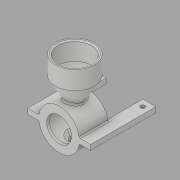
# Autodesk Inventor part: powderTurnRes
Saved by Autodesk Inventor 2017 (Build 210142000, 142)
## iProperties
Created: 2019-05-09
Part Number: powderTurnRes
Material: Generic
Document SubType Name: Modeling
Designer: Joe Sedutto
Density: 1 g/cm^3
Appearance: Default
Author: Joe Sedutto
Autodesk Inventor part; units mm, degrees
ref_plane "YZ Plane" through (0, 0, 0) normal (1, 0, 0) x (0, 1, 0)
ref_plane "XY Plane" through (0, 0, 0) normal (0, 0, 1) x (1, 0, 0)
sketch "Sketch1" plane through (0, 0, 0) normal (0, 0, 1) x (1, 0, 0)
  circle A0 centre (0, 0) radius 13.335
  circle A1 centre (0, 0) radius 19.685
  dimension "d0" = 26.67
  dimension "d1" = 6.35
  constraints: 2 centre point, 1 coincident
  measures "d0" diameter of A0
  measures "d1" radial gap between concentric circles of A0 A1
extrude "Extrusion1" add sketch "Sketch1" along normal blind 25.4
sketch "Sketch2" plane through (0, 0, 25.4) normal (0, 0, 1) x (1, 0, 0)
  circle A0 centre (0, 0) radius 13.335 projected
  circle A1 centre (0, 0) radius 19.685 projected
  circle A2 centre (0, 0) radius 12.065
  dimension "d4" = 1.27
  constraints: 1 centre point
  measures "d4" radial gap between concentric circles of A0 A2
extrude "Extrusion2" add sketch "Sketch2" along normal blind 2.54 contours A0 | A1
ref_plane "Work Plane1" through (0, 19.685, 0) normal (0, 1, 0) x (-1, 0, 0)
sketch "Sketch3" plane through (0, 19.685, 0) normal (0, 1, 0) x (-1, 0, 0)
  line L0 (-13.335, 0) -> (-13.335, 25.4) projected
  line L1 (0, 12.7) -> (-13.335, 12.7) construction
  line L2 (13.335, 0) -> (13.335, 25.4) projected
  line L3 (13.335, 12.7) -> (0, 12.7) construction
  point P0 (0, 0)
  constraints: 4 end point, 2 midpoint, 1 collinear, 1 horizontal
hole "Hole1" at (0, 19.685, 12.7) direction (0, -1, 0) diameter 6.35 depth 12.7 tip angle 118
ref_plane "Work Plane2" through (0, 0, 12.7) normal (0, 0, -1) x (-1, 0, 0)
sketch "Sketch4" plane through (0, 0, 12.7) normal (0, 0, -1) x (-1, 0, 0)
  line L0 (-3.175, 15.4915) -> (-16.228, 38.1)
  line L1 (-16.228, 38.1) -> (-18.768, 38.1)
  line L2 (-18.768, 38.1) -> (-5.715, 15.4915)
  line L3 (-5.715, 15.4915) -> (-3.175, 15.4915)
  circle A0 centre (0, 0) radius 19.685 projected
  line L4 (0, 19.685) -> (0, 34.1207) construction
  line L5 (-3.175, 12.9515) -> (-3.175, 19.4273) projected
  dimension "d15" = 2.54
  dimension "d16" = 38.1
  dimension "d17" = 30
  dimension "d18" = 2.54
  constraints: 10 end point, 2 parallel, 1 horizontal, 1 point on circle, 1 point on line, 1 vertical
  measures "d15" distance of L0.end L1.end
  measures "d16" distance from line of L1 point (0, 0)
  measures "d17" angle of L4 L2
  measures "d18" distance of L0.start L5.start
revolve "Revolution1" add sketch "Sketch4" angle 360 about axis through (0, 19.685, 12.7) along (0, 1, 0) contours L3 L2 A0 L0 | A0 L2 L1 L0
sketch "Sketch5" plane through (0, 38.1, 12.7) normal (0, 1, 0) x (1, 0, 0)
  circle A0 centre (0, 0) radius 18.768 projected
  circle A1 centre (0, 0) radius 16.228 projected
  point P0 (0, 12.7)
extrude "Extrusion3" add sketch "Sketch5" along normal blind 17.78
fillet "Fillet1" radius 1.27 1 edges at (-16.228, 55.88, 12.7)
fillet "Fillet2" radius 1.27 1 edges at (-7.3209, 18.273, 12.6991)
sketch "Sketch7" plane through (0, 0, 0) normal (0, 1, 0) x (-1, 0, 0)
  spline S0 degree 5 poles (0, 15.875) (0.3658, 15.875) (0.7269, 15.8223) (1.0689, 15.7198) (1.3811, 15.5769) (2.0115, 15.1917) (2.3108, 14.9286) (2.5556, 14.6369) (2.7488, 14.3276) (3.1275, 13.4883) (3.2362, 12.9391) (3.2299, 12.3842) (3.108, 11.8361) (2.6851, 10.9581) (2.4466, 10.6105) (2.1388, 10.2882) (1.7587, 10.0103) (0.8989, 9.6224) (0.4259, 9.4951) (-0.0811, 9.4669) (-0.5724, 9.5429) (-1.4458, 9.8363) (-1.8264, 10.0514) (-2.1489, 10.3127) (-2.4131, 10.6031) (-2.8482, 11.2413) (-3.0127, 11.5938) (-3.1209, 11.9589) (-3.175, 12.3292) (-3.175, 13.0561) (-3.1251, 13.4117) (-3.0253, 13.7627) (-2.8738, 14.1025) (-2.4642, 14.7367) (-2.2072, 15.0334) (-1.8916, 15.3023) (-1.5168, 15.5267) (-0.8852, 15.7566) (-0.6727, 15.8148) (-0.4518, 15.8549) (-0.2262, 15.875) (0, 15.875) knots 0 0 0 0 0 0 0.075674 0.075674 0.075674 0.075674 0.173825 0.173825 0.173825 0.173825 0.331664 0.331664 0.331664 0.331664 0.443615 0.443615 0.443615 0.443615 0.544209 0.544209 0.544209 0.544209 0.643845 0.643845 0.643845 0.643845 0.750428 0.750428 0.750428 0.750428 0.852775 0.852775 0.852775 0.852775 0.953216 0.953216 0.953216 0.953216 1 1 1 1 1 1
  spline S1 degree 5 poles (0, 17.145) (1.3934, 17.1441) (2.7891, 16.6018) (3.8921, 15.4994) (4.9888, 12.7159) (3.9096, 9.9248) (2.813, 8.8173) (0.0263, 7.709) (-2.7752, 8.7855) (-3.8891, 9.8896) (-4.9935, 12.6868) (-3.9033, 15.488) (-2.7986, 16.5982) (-1.3982, 17.1441) (0, 17.145) knots 0 0 0 0 0 0 0.249522 0.249522 0.249522 0.498935 0.498935 0.498935 0.749627 0.749627 0.749627 1 1 1 1 1 1
  point P0 (0, 0)
  dimension "d30" = 1.27
  constraints: 3 other
extrude "Extrusion5" cut sketch "Sketch7" against normal blind 25.4 contours S0 | S1
chamfer "Chamfer2" distance 3.175 angle 45 1 edges at (0.0013, -13.335, 8.2552)
sketch "Sketch8" plane through (0, 0, 0) normal (0, 1, 0) x (-1, 0, 0)
  line L0 (19.685, 27.94) -> (-19.685, 27.94) projected
  line L1 (17.78, 27.94) -> (30.48, 27.94)
  line L2 (30.48, 27.94) -> (30.48, -35.56)
  line L3 (30.48, -35.56) -> (17.78, -35.56)
  line L4 (17.78, -35.56) -> (17.78, 27.94)
  line L5 (0, 27.94) -> (0, -6.068) construction
  circle A0 centre (0, 12.7) radius 18.768 projected
  line L6 (-19.685, 27.94) -> (19.685, 27.94)
  line L7 (-17.78, 27.94) -> (-30.48, 27.94)
  line L8 (-30.48, 27.94) -> (-30.48, -35.56)
  line L9 (-30.48, -35.56) -> (-17.78, -35.56)
  line L10 (-17.78, -35.56) -> (-17.78, 27.94)
  circle A1 centre (0, 12.7) radius 18.768
  point P0 (0, 0)
  dimension "d36" = 12.7
  dimension "d37" = 17.78
  dimension "d38" = 63.5
  constraints: 20 end point, 6 symmetric about line, 2 parallel, 2 point on line, 1 centre point, 1 horizontal, 1 line through centre, 1 midpoint, 1 perpendicular, 1 vertical, 1 vertical alignment, 1 other
  measures "d36" distance between parallel lines of L4 L2
  measures "d37" distance from line of A1.centre L4
  measures "d38" distance between parallel lines of L1 L3
extrude "Extrusion6" add sketch "Sketch8" along normal mid plane 5.08 contours L1 L2 L3 L4 A0 L0 | A0 L4 | L10 A0 L9 L8 L7 L0 | L10 A0
fillet "Fillet3" radius 1.27 4 edges at (19.5204, 2.54, 13.97) (-19.5204, 2.54, 13.97) (-19.5204, -2.54, 13.97) (19.5204, -2.54, 13.97)
sketch "Sketch9" plane through (0, 2.54, 0) normal (0, 1, 0) x (1, 0, 0)
  line L0 (17.78, 35.56) -> (17.78, 0) projected
  line L1 (30.48, 35.56) -> (17.78, 35.56)
  line L2 (17.78, 35.56) -> (17.78, 22.86)
  line L3 (17.78, 22.86) -> (30.48, 22.86)
  line L4 (30.48, 22.86) -> (30.48, 35.56)
  line L5 (30.48, 35.56) -> (17.78, 22.86) construction
  line L6 (17.78, 35.56) -> (30.48, 22.86) construction
  line L7 (-30.48, -27.94) -> (-30.48, 35.56) projected
  line L8 (-17.78, 35.56) -> (-30.48, 35.56)
  line L9 (-30.48, 35.56) -> (-30.48, 22.86)
  line L10 (-30.48, 22.86) -> (-17.78, 22.86)
  line L11 (-17.78, 22.86) -> (-17.78, 35.56)
  line L12 (-17.78, 35.56) -> (-30.48, 22.86) construction
  line L13 (-30.48, 35.56) -> (-17.78, 22.86) construction
  line L14 (30.48, 35.56) -> (17.78, 35.56) projected
  line L15 (30.48, -27.94) -> (30.48, 35.56) projected
  line L16 (-17.78, 35.56) -> (-30.48, 35.56) projected
  line L17 (-17.78, 0) -> (-17.78, 35.56) projected
  point P0 (0, 0)
  point P1 (24.13, 29.21)
  point P2 (-24.13, 29.21)
  point P3 (24.13, 29.21)
  point P4 (-24.13, 29.21)
  constraints: 24 end point, 4 collinear, 4 midpoint, 4 parallel, 3 perpendicular, 3 point on line, 2 coincident, 2 horizontal
hole "Hole2" at (24.13, 2.54, -29.21) at (-24.13, 2.54, -29.21) direction (0, -1, 0) diameter 4.2333 depth 12.7 tip angle 118
body "Solid1"
